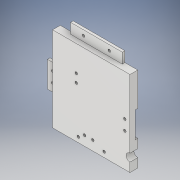
# Autodesk Inventor part: CP007
Saved by Autodesk Inventor 2017 SP1 (Build 210196100, 196)
## iProperties
Created: 2017-05-15
Part Number: CP007
Material: ABS Plastic
Document SubType Name: Modeling
Designer: zallen
Density: 1.06 g/cm^3
Appearance: Smooth - White
Mass: 391.263 g
Surface Area: 662.381 cm^2
Volume: 369.116 cm^3
Author: zallen
Autodesk Inventor part; units mm, degrees
ref_plane "YZ Plane" through (0, 0, 0) normal (1, 0, 0) x (0, 1, 0)
ref_plane "XZ Plane" through (0, 0, 0) normal (0, 1, 0) x (-1, 0, 0)
ref_plane "XY Plane" through (0, 0, 0) normal (0, 0, 1) x (1, 0, 0)
sketch "Sketch1" plane through (0, 0, 0) normal (0, 0, 1) x (1, 0, 0)
  line L0 (0, 0) -> (150, 0)
  line L1 (150, 0) -> (150, 164.5751)
  line L2 (150, 164.5751) -> (0, 164.5751)
  line L3 (0, 164.5751) -> (0, 0)
  dimension "d0" = 150
  dimension "d1" = 164.5751
  constraints: 8 end point, 2 parallel, 1 horizontal, 1 perpendicular
  measures "d0" distance of L2.end L1.end
  measures "d1" distance of L1.end L0.end
extrude "Extrusion1" add sketch "Sketch1" along normal blind 15
sketch "Sketch7" plane through (0, 0, 0) normal (0, 0, -1) x (-1, 0, 0)
  line L0 (0, 50) -> (20, 50)
  line L1 (20, 50) -> (20, 100)
  line L2 (20, 100) -> (0, 100)
  line L3 (0, 100) -> (0, 50)
  point P0 (0, 0)
  dimension "d27" = 20
  dimension "d28" = 50
  dimension "d29" = 50
  constraints: 8 end point, 2 parallel, 1 horizontal, 1 perpendicular
  measures "d27" distance of L2.end L1.end
  measures "d28" distance of L1.end L0.end
  measures "d29" distance of point (0, 0) L0.start
extrude "Extrusion7" add sketch "Sketch7" against normal blind 5
sketch "Sketch8" plane through (0, 0, 0) normal (0, 0, -1) x (-1, 0, 0)
  line L0 (-150, 164.5751) -> (0, 164.5751) projected
  line L1 (-25, 164.5751) -> (-125, 164.5751)
  line L2 (-125, 164.5751) -> (-125, 184.5751)
  line L3 (-125, 184.5751) -> (-25, 184.5751)
  line L4 (-25, 184.5751) -> (-25, 164.5751)
  point P0 (0, 0)
  dimension "d37" = 100
  dimension "d38" = 20
  constraints: 8 end point, 2 parallel, 1 horizontal, 1 perpendicular, 1 point on line
  measures "d37" distance of L2.end L3.end
  measures "d38" distance of L1.end L2.end
extrude "Extrusion8" add sketch "Sketch8" against normal blind 5
sketch "Sketch9" plane through (0, 0, 0) normal (0, 0, -1) x (-1, 0, 0)
  circle A0 centre (-50, 174.5751) radius 2.5
  circle A1 centre (-100, 174.5751) radius 2.5
  line L0 (-125, 184.5751) -> (-25, 184.5751) projected
  circle A2 centre (10, 65) radius 2.5
  circle A3 centre (10, 85) radius 2.5
  line L1 (0, 100) -> (0, 50) projected
  line L2 (0, 50) -> (20, 50) projected
  line L3 (20, 100) -> (0, 100) projected
  point P0 (0, 0)
  dimension "d44" = 5
  dimension "d45" = 5
  dimension "d46" = 10
  dimension "d47" = 5
  dimension "d48" = 5
  dimension "d49" = 10
  dimension "d50" = 15
  dimension "d51" = 15
  constraints: 4 centre point, 1 horizontal alignment, 1 vertical alignment
  measures "d44" diameter of A0
  measures "d45" diameter of A1
  measures "d46" distance from line of L0 A0.centre
  measures "d47" diameter of A2
  measures "d48" diameter of A3
  measures "d49" distance from line of L1 A2.centre
  measures "d50" distance from line of L2 A2.centre
  measures "d51" distance from line of L3 A3.centre
extrude "Extrusion9" cut sketch "Sketch9" against normal through all
thread "Thread1" size "M5x0.8" class "6H" standard "ANSI Metric M Profile" full length
thread "Thread2" size "M5x0.8" class "6H" standard "ANSI Metric M Profile" full length
thread "Thread3" size "M5x0.8" class "6H" standard "ANSI Metric M Profile" full length
thread "Thread4" size "M5x0.8" class "6H" standard "ANSI Metric M Profile" full length
sketch "Sketch10" plane through (0, 0, 0) normal (0, 0, -1) x (-1, 0, 0)
  line L0 (-150, 0) -> (-150, 164.5751) projected
  line L1 (-150, 50) -> (-130, 50)
  line L2 (-130, 50) -> (-130, 100)
  line L3 (-130, 100) -> (-150, 100)
  line L4 (-150, 100) -> (-150, 50)
  line L5 (0, 0) -> (-150, 0) projected
  line L6 (0, 50) -> (0, 0) projected
  line L7 (0, 50) -> (20, 50) projected
  line L8 (20, 50) -> (20, 100) projected
  line L9 (20, 100) -> (0, 100) projected
  line L10 (0, 164.5751) -> (0, 100) projected
  line L11 (-25, 164.5751) -> (0, 164.5751) projected
  line L12 (-150, 0) -> (-150, 164.5751) projected
  line L13 (-25, 184.5751) -> (-25, 164.5751) projected
  line L14 (-125, 184.5751) -> (-25, 184.5751) projected
  line L15 (-125, 164.5751) -> (-125, 184.5751) projected
  line L16 (-150, 164.5751) -> (-125, 164.5751) projected
  dimension "d66" = 20
  dimension "d67" = 50
  constraints: 8 end point, 2 parallel, 1 horizontal, 1 horizontal alignment, 1 perpendicular, 1 point on line
  measures "d66" distance of L3.end L2.end
  measures "d67" distance of L2.end L1.end
extrude "Extrusion10" cut sketch "Sketch10" against normal blind 5 contours L0 L3 L2 L1
sketch "Sketch11" plane through (0, 0, 5) normal (0, 0, -1) x (-1, 0, 0)
  circle A0 centre (-140, 85) radius 2.5
  circle A1 centre (-140, 65) radius 2.5
  line L0 (-130, 50) -> (-150, 50) projected
  line L1 (-150, 0) -> (-150, 50) projected
  line L2 (0, 0) -> (-150, 0) projected
  line L3 (0, 50) -> (0, 0) projected
  line L4 (0, 50) -> (20, 50) projected
  line L5 (20, 50) -> (20, 100) projected
  line L6 (20, 100) -> (0, 100) projected
  line L7 (0, 164.5751) -> (0, 100) projected
  line L8 (-25, 164.5751) -> (0, 164.5751) projected
  line L9 (-150, 100) -> (-150, 164.5751) projected
  line L10 (-150, 100) -> (-130, 100) projected
  line L11 (-130, 100) -> (-130, 50) projected
  line L12 (-150, 50) -> (-150, 100) projected
  line L13 (-25, 184.5751) -> (-25, 164.5751) projected
  line L14 (-125, 184.5751) -> (-25, 184.5751) projected
  line L15 (-125, 164.5751) -> (-125, 184.5751) projected
  line L16 (-150, 164.5751) -> (-125, 164.5751) projected
  dimension "d70" = 5
  dimension "d71" = 5
  dimension "d72" = 10
  dimension "d96" = 15
  dimension "d97" = 15
  constraints: 2 centre point, 1 vertical alignment
  measures "d70" diameter of A0
  measures "d71" diameter of A1
  measures "d72" distance from line of L12 A1.centre
  measures "d96" distance from line of L10 A0.centre
  measures "d97" distance from line of L0 A1.centre
extrude "Extrusion11" cut sketch "Sketch11" against normal through all contours A0 | A1
thread "Thread7" size "M5x0.8" class "6H" standard "ANSI Metric M Profile" full length
thread "Thread8" size "M5x0.8" class "6H" standard "ANSI Metric M Profile" full length
sketch "Sketch12" plane through (0, 0, 0) normal (0, 0, -1) x (-1, 0, 0)
  line L0 (0, 0) -> (-150, 0) projected
  line L1 (-25, 0) -> (-125, 0)
  line L2 (-125, 0) -> (-125, 20)
  line L3 (-125, 20) -> (-25, 20)
  line L4 (-25, 20) -> (-25, 0)
  dimension "d79" = 100
  dimension "d80" = 20
  dimension "d81" = 25
  constraints: 8 end point, 2 parallel, 1 horizontal, 1 perpendicular, 1 point on line
  measures "d79" distance of L2.end L3.end
  measures "d80" distance of L1.end L2.end
  measures "d81" distance from line of L0.start L4
extrude "Extrusion12" cut sketch "Sketch12" against normal blind 5
sketch "Sketch13" plane through (0, 0, 5) normal (0, 0, -1) x (-1, 0, 0)
  circle A0 centre (-50, 10) radius 2.5
  circle A1 centre (-100, 10) radius 2.5
  line L0 (-25, 20) -> (-25, 0) projected
  line L1 (-125, 0) -> (-125, 20) projected
  line L2 (-125, 20) -> (-25, 20) projected
  point P0 (0, 0)
  dimension "d84" = 5
  dimension "d85" = 5
  dimension "d86" = 25
  dimension "d87" = 25
  dimension "d88" = 10
  dimension "d89" = 10
  constraints: 2 centre point
  measures "d84" diameter of A0
  measures "d85" diameter of A1
  measures "d86" distance from line of A0.centre L0
  measures "d87" distance from line of L1 A1.centre
  measures "d88" distance from line of L2 A0.centre
  measures "d89" distance from line of L2 A1.centre
extrude "Extrusion13" cut sketch "Sketch13" against normal through all
thread "Thread9" size "M5x0.8" class "6H" standard "ANSI Metric M Profile" full length
thread "Thread10" size "M5x0.8" class "6H" standard "ANSI Metric M Profile" full length
sketch "Sketch14" plane through (0, 0, 0) normal (0, 0, -1) x (-1, 0, 0)
  circle A0 centre (-46, 98.5751) radius 2.5
  circle A1 centre (-46, 114.5751) radius 2.5
  line L0 (-150, 0) -> (-150, 50) projected
  line L1 (-25, 164.5751) -> (0, 164.5751) projected
  point P0 (0, 0)
  dimension "d98" = 5
  dimension "d99" = 5
  dimension "d100" = 104
  dimension "d101" = 16
  dimension "d112" = 50
  constraints: 2 centre point, 1 vertical alignment
  measures "d98" diameter of A0
  measures "d99" diameter of A1
  measures "d100" distance from line of L0 A0.centre
  measures "d101" distance of A1.centre A0.centre
  measures "d112" distance from line of L1 A1.centre
extrude "Extrusion14" cut sketch "Sketch14" against normal through all
thread "Thread11" size "M5x0.8" class "6H" standard "ANSI Metric M Profile" full length
thread "Thread12" size "M5x0.8" class "6H" standard "ANSI Metric M Profile" full length
sketch "Sketch15" plane through (0, 0, 0) normal (0, 0, -1) x (-1, 0, 0)
  line L0 (0, 50) -> (0, 0) construction
  line L1 (0, 25) -> (-166.3401, 25) construction
  line L2 (-150, 0) -> (-150, 164.5751) projected
  circle A0 centre (-150, 25) radius 7.5
  dimension "d109" = 15
  constraints: 2 end point, 2 point on line, 1 centre point, 1 horizontal, 1 midpoint
  measures "d109" diameter of A0
extrude "Extrusion15" cut sketch "Sketch15" against normal through all
sketch "Sketch16" plane through (0, 0, 15) normal (0, 0, 1) x (1, 0, 0)
  circle A0 centre (62, 18.5751) radius 2.5
  circle A1 centre (78, 18.5751) radius 2.5
  circle A2 centre (46, 98.5751) radius 2.5 projected
  circle A3 centre (46, 114.5751) radius 2.5 projected
  point P0 (0, 0)
  dimension "d113" = 5
  dimension "d114" = 5
  dimension "d115" = 16
  dimension "d116" = 80
  dimension "d117" = 16
  constraints: 2 centre point, 1 horizontal alignment
  measures "d113" diameter of A0
  measures "d114" diameter of A1
  measures "d115" distance of A1.centre A0.centre
  measures "d116" vertical distance of A0.centre A2.centre
  measures "d117" horizontal distance of A0.centre A2.centre
extrude "Extrusion16" cut sketch "Sketch16" against normal blind 5 contours A0 | A1
thread "Thread13" size "M5x0.8" class "6H" standard "ANSI Metric M Profile" full length
thread "Thread14" size "M5x0.8" class "6H" standard "ANSI Metric M Profile" full length
body "Solid1"
